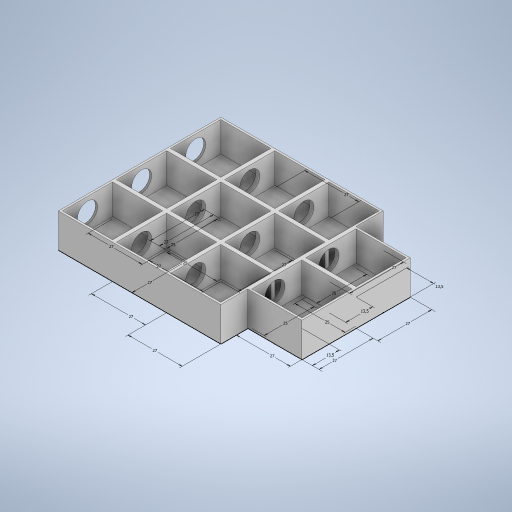
# Autodesk Inventor part: новая коробка
Saved by Autodesk Inventor 2024.2 (Build 282272000, 272)
## iProperties
Created: 2026-01-06
Part Number: новая коробка
Material: Типовые
Document SubType Name: Modeling
Designer: User
Density: 1 g/cm^3
Appearance: По умолчанию
Author: User
Autodesk Inventor part; units mm, degrees
ref_plane "YZ Plane" through (0, 0, 0) normal (1, 0, 0) x (0, 1, 0)
ref_plane "XZ Plane" through (0, 0, 0) normal (0, 1, 0) x (-1, 0, 0)
ref_plane "XY Plane" through (0, 0, 0) normal (0, 0, 1) x (1, 0, 0)
sketch "Эскиз1" plane through (0, 0, 0) normal (0, 1, 0) x (-1, 0, 0)
  line L0 (-12.5, -12.5) -> (12.5, -12.5)
  line L1 (12.5, -12.5) -> (12.5, 12.5)
  line L2 (12.5, 12.5) -> (-12.5, 12.5)
  line L3 (-12.5, 12.5) -> (-12.5, -12.5)
  line L4 (-12.5, -12.5) -> (12.5, 12.5) construction
  line L5 (12.5, -12.5) -> (-12.5, 12.5) construction
  line L6 (-13.5, -13.5) -> (13.5, -13.5)
  line L7 (13.5, -13.5) -> (13.5, 13.5)
  line L8 (13.5, 13.5) -> (-13.5, 13.5)
  line L9 (-13.5, 13.5) -> (-13.5, -13.5)
  line L10 (-13.5, -13.5) -> (13.5, 13.5) construction
  line L11 (13.5, -13.5) -> (-13.5, 13.5) construction
  line L12 (13.5, 13.5) -> (40.5, 13.5)
  line L13 (40.5, 13.5) -> (40.5, -13.5)
  line L14 (40.5, -13.5) -> (13.5, -13.5)
  line L15 (13.5, -13.5) -> (13.5, 13.5)
  line L16 (-13.5, 13.5) -> (-40.5, 13.5)
  line L17 (-40.5, 13.5) -> (-40.5, -13.5)
  line L18 (-40.5, -13.5) -> (-13.5, -13.5)
  line L19 (-13.5, -13.5) -> (-13.5, 13.5)
  line L20 (40.5, -13.5) -> (13.5, -13.5)
  line L21 (13.5, -13.5) -> (13.5, -40.5)
  line L22 (13.5, -40.5) -> (40.5, -40.5)
  line L23 (40.5, -40.5) -> (40.5, -13.5)
  line L24 (-13.5, -13.5) -> (13.5, -13.5)
  line L25 (13.5, -13.5) -> (13.5, -40.5)
  line L26 (13.5, -40.5) -> (-13.5, -40.5)
  line L27 (-13.5, -40.5) -> (-13.5, -13.5)
  line L28 (-13.5, -13.5) -> (-40.5, -13.5)
  line L29 (-40.5, -13.5) -> (-40.5, -40.5)
  line L30 (-40.5, -40.5) -> (-13.5, -40.5)
  line L31 (-13.5, -40.5) -> (-13.5, -13.5)
  line L32 (40.5, 13.5) -> (13.5, 13.5)
  line L33 (13.5, 13.5) -> (13.5, 40.5)
  line L34 (13.5, 40.5) -> (40.5, 40.5)
  line L35 (40.5, 40.5) -> (40.5, 13.5)
  line L36 (13.5, 40.5) -> (-13.5, 40.5)
  line L37 (-13.5, 40.5) -> (-13.5, 13.5)
  line L38 (-13.5, 13.5) -> (13.5, 13.5)
  line L39 (13.5, 13.5) -> (13.5, 40.5)
  line L40 (-13.5, 40.5) -> (-40.5, 40.5)
  line L41 (-40.5, 40.5) -> (-40.5, 13.5)
  line L42 (-40.5, 13.5) -> (-13.5, 13.5)
  line L43 (-13.5, 13.5) -> (-13.5, 40.5)
  line L44 (-40.5, 0) -> (-67.5, 0)
  line L45 (-67.5, 0) -> (-67.5, -27)
  line L46 (-67.5, -27) -> (-40.5, -27)
  line L47 (-40.5, -27) -> (-40.5, 0)
  line L48 (-40.5, 0) -> (-67.5, 0)
  line L49 (-67.5, 0) -> (-67.5, 27)
  line L50 (-67.5, 27) -> (-40.5, 27)
  line L51 (-40.5, 27) -> (-40.5, 0)
  line L52 (-12.5, 14.5) -> (12.5, 14.5)
  line L53 (12.5, 14.5) -> (12.5, 39.5)
  line L54 (12.5, 39.5) -> (-12.5, 39.5)
  line L55 (-12.5, 39.5) -> (-12.5, 14.5)
  line L56 (-12.5, 14.5) -> (12.5, 39.5) construction
  line L57 (12.5, 14.5) -> (-12.5, 39.5) construction
  line L58 (14.5, 14.5) -> (39.5, 14.5)
  line L59 (39.5, 14.5) -> (39.5, 39.5)
  line L60 (39.5, 39.5) -> (14.5, 39.5)
  line L61 (14.5, 39.5) -> (14.5, 14.5)
  line L62 (14.5, 14.5) -> (39.5, 39.5) construction
  line L63 (39.5, 14.5) -> (14.5, 39.5) construction
  line L64 (-39.5, 14.5) -> (-14.5, 14.5)
  line L65 (-14.5, 14.5) -> (-14.5, 39.5)
  line L66 (-14.5, 39.5) -> (-39.5, 39.5)
  line L67 (-39.5, 39.5) -> (-39.5, 14.5)
  line L68 (-39.5, 14.5) -> (-14.5, 39.5) construction
  line L69 (-14.5, 14.5) -> (-39.5, 39.5) construction
  line L70 (-39.5, -12.5) -> (-14.5, -12.5)
  line L71 (-14.5, -12.5) -> (-14.5, 12.5)
  line L72 (-14.5, 12.5) -> (-39.5, 12.5)
  line L73 (-39.5, 12.5) -> (-39.5, -12.5)
  line L74 (-39.5, -12.5) -> (-14.5, 12.5) construction
  line L75 (-14.5, -12.5) -> (-39.5, 12.5) construction
  line L76 (-39.5, -39.5) -> (-14.5, -39.5)
  line L77 (-14.5, -39.5) -> (-14.5, -14.5)
  line L78 (-14.5, -14.5) -> (-39.5, -14.5)
  line L79 (-39.5, -14.5) -> (-39.5, -39.5)
  line L80 (-39.5, -39.5) -> (-14.5, -14.5) construction
  line L81 (-14.5, -39.5) -> (-39.5, -14.5) construction
  line L82 (14.5, -39.5) -> (39.5, -39.5)
  line L83 (39.5, -39.5) -> (39.5, -14.5)
  line L84 (39.5, -14.5) -> (14.5, -14.5)
  line L85 (14.5, -14.5) -> (14.5, -39.5)
  line L86 (14.5, -39.5) -> (39.5, -14.5) construction
  line L87 (39.5, -39.5) -> (14.5, -14.5) construction
  line L88 (-12.5, -39.5) -> (12.5, -39.5)
  line L89 (12.5, -39.5) -> (12.5, -14.5)
  line L90 (12.5, -14.5) -> (-12.5, -14.5)
  line L91 (-12.5, -14.5) -> (-12.5, -39.5)
  line L92 (-12.5, -39.5) -> (12.5, -14.5) construction
  line L93 (12.5, -39.5) -> (-12.5, -14.5) construction
  line L94 (14.5, -12.5) -> (39.5, -12.5)
  line L95 (39.5, -12.5) -> (39.5, 12.5)
  line L96 (39.5, 12.5) -> (14.5, 12.5)
  line L97 (14.5, 12.5) -> (14.5, -12.5)
  line L98 (14.5, -12.5) -> (39.5, 12.5) construction
  line L99 (39.5, -12.5) -> (14.5, 12.5) construction
  line L100 (-66.5, -26) -> (-41.5, -26)
  line L101 (-41.5, -26) -> (-41.5, -1)
  line L102 (-41.5, -1) -> (-66.5, -1)
  line L103 (-66.5, -1) -> (-66.5, -26)
  line L104 (-66.5, -26) -> (-41.5, -1) construction
  line L105 (-41.5, -26) -> (-66.5, -1) construction
  line L106 (-66.5, 26) -> (-41.5, 26)
  line L107 (-41.5, 26) -> (-41.5, 1)
  line L108 (-41.5, 1) -> (-66.5, 1)
  line L109 (-66.5, 1) -> (-66.5, 26)
  line L110 (-66.5, 26) -> (-41.5, 1) construction
  line L111 (-41.5, 26) -> (-66.5, 1) construction
  point P0 (0, 0)
  point P1 (0, 27)
  point P2 (27, 27)
  point P3 (-27, 27)
  point P4 (-27, 0)
  point P5 (-27, -27)
  point P6 (27, -27)
  point P7 (0, -27)
  point P8 (27, 0)
  point P9 (-54, -13.5)
  point P10 (-54, 0)
  point P11 (-67.5, -13.5)
  point P12 (-54, 13.5)
  point P13 (-54, 27)
  dimension "d0" = 25
  dimension "d1" = 25
  dimension "d2" = 27
  dimension "d3" = 27
  dimension "d4" = 27
  dimension "d5" = 27
  dimension "d6" = 27
  dimension "d7" = 27
  dimension "d8" = 27
  dimension "d9" = 27
  dimension "d10" = 27
  dimension "d11" = 27
  dimension "d12" = 27
  dimension "d13" = 27
  dimension "d14" = 27
  dimension "d15" = 25
  dimension "d16" = 25
  dimension "d17" = 13.5
  dimension "d18" = 13.5
  dimension "d19" = 25
  dimension "d20" = 13.5
  constraints: 224 end point, 44 parallel, 28 midpoint, 22 horizontal, 22 perpendicular, 15 point on line
  measures "d0" distance of L0.end L1.end
  measures "d1" distance of L1.end L2.end
  measures "d2" distance of L6.end L7.end
  measures "d3" distance of L7.end L8.end
  measures "d4" distance of L7.end L12.end
  measures "d5" distance of L32.end L33.end
  measures "d6" distance of L49.end L50.end
  measures "d7" distance of L36.end L40.end
  measures "d8" distance of L33.end L36.end
  measures "d9" distance of L21.end L26.end
  measures "d10" distance of L28.end L29.end
  measures "d11" distance of L48.end L49.end
  measures "d12" distance of L44.end L45.end
  measures "d13" distance of L14.end L7.end
  measures "d14" distance of L18.end L8.end
  measures "d15" distance of L100.end L101.end
  measures "d16" distance of L101.end L102.end
  measures "d17" distance of point (-54, 0) point (-54, -13.5)
  measures "d18" distance of point (-67.5, -13.5) point (-54, -13.5)
  measures "d19" distance of L106.end L107.end
  measures "d20" distance of point (-54, 27) point (-54, 13.5)
extrude "Выдавливание1" add sketch "Эскиз1" along normal blind 17
extrude "Выдавливание2" add sketch "Эскиз1" along normal blind 2 contours L3 L2 L1 L0 | L55 L54 L53 L52 | L61 L60 L59 L58 | L67 L66 L65 L64 | L73 L72 L71 L70 | L79 L78 L77 L76 | L85 L84 L83 L82 | L91 L90 L89 L88 | L97 L96 L95 L94 | L103 L102 L101 L100 | L106 L107 L108 L109
sketch "Эскиз2" plane through (-39.5, 17, 39.5) normal (1, 0, 0) x (0, 0, -1)
  line L0 (0, -15) -> (25, -15) projected
  line L1 (25, -15) -> (25, 0) projected
  line L2 (0, 0) -> (25, 0) projected
  line L3 (0, -15) -> (0, 0) projected
  line L4 (27, -15) -> (52, -15) projected
  line L5 (52, -15) -> (52, 0) projected
  line L6 (27, 0) -> (52, 0) projected
  line L7 (27, -15) -> (27, 0) projected
  line L8 (54, -15) -> (79, -15) projected
  line L9 (79, -15) -> (79, 0) projected
  line L10 (54, 0) -> (79, 0) projected
  line L11 (54, -15) -> (54, 0) projected
  circle A0 centre (12.5, -7) radius 5
  line L12 (0, -15) -> (25, -15) projected
  circle A1 centre (39.5, -7) radius 5
  circle A2 centre (66.5, -7) radius 5
  line L13 (27, -15) -> (52, -15) projected
  point P0 (39.5, -17)
  point P1 (12.5, -15)
  point P2 (39.5, -15)
  dimension "d25" = 10
  dimension "d26" = 8
  dimension "d27" = 10
  dimension "d28" = 10
  dimension "d29" = 8
  dimension "d30" = 8
  constraints: 3 centre point, 2 midpoint
  measures "d25" diameter of A0
  measures "d26" distance of point (12.5, -15) A0.centre
  measures "d27" diameter of A1
  measures "d28" diameter of A2
  measures "d29" distance of point (39.5, -15) A1.centre
  measures "d30" distance from line of L8 A2.centre
extrude "Выдавливание3" cut sketch "Эскиз2" along normal blind 70 and the other way blind 35 contours A0 | A1 | A2
sketch "Эскиз3" plane through (41.5, 17, 26) normal (1, 0, 0) x (0, 0, -1)
  line L0 (11.5, -15) -> (11.5, 0) projected
  circle A0 centre (11.5, -7) radius 5
  line L1 (38.5, -15) -> (38.5, 0) projected
  circle A1 centre (38.5, -7) radius 5
  point P0 (26, -17)
  dimension "d35" = 10
  dimension "d36" = 8
  dimension "d37" = 10
  dimension "d38" = 8
  constraints: 2 centre point, 2 point on line
  measures "d35" diameter of A0
  measures "d36" distance of A0.centre L0.start
  measures "d37" diameter of A1
  measures "d38" distance of A1.centre L1.start
extrude "Выдавливание4" cut sketch "Эскиз3" against normal blind 2
